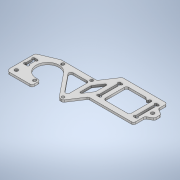
# Autodesk Inventor part: Ankle_side_frame
Saved by Autodesk Inventor 2020.4 (Build 244396000, 396)
## iProperties
Part Number: Ankle_side_frame
Material: アルミニウム 2014-T4
Document SubType Name: Modeling
Designer: Masato Kubotera
Density: 2.8 g/cm^3
Appearance: 滑らか - 淡い灰色
Description: A2017 T2
Mass: 9.74724 g
Surface Area: 49.2982 cm^2
Volume: 3.48116 cm^3
Author: Masato Kubotera
Autodesk Inventor part; units mm, degrees
ref_plane "YZ Plane" through (0, 0, 0) normal (1, 0, 0) x (0, 1, 0)
ref_plane "XZ Plane" through (0, 0, 0) normal (0, 1, 0) x (-1, 0, 0)
ref_plane "XY Plane" through (0, 0, 0) normal (0, 0, 1) x (1, 0, 0)
sketch "スケッチ1" plane through (0, 0, 0) normal (0, 0, 1) x (1, 0, 0)
  line L0 (28, 13.5) -> (1, 13.5) construction
  line L1 (1, 13.5) -> (1, -13.5) construction
  line L2 (1, -13.5) -> (28, -13.5) construction
  line L3 (28, -13.5) -> (28, 13.5) construction
  line L4 (28, 13.5) -> (1, -13.5) construction
  line L5 (1, 13.5) -> (28, -13.5) construction
  circle A0 centre (0, 0) radius 10.5 construction
  arc A1 (0, 16) -> (-12, 10.583) centre (0, 0) ccw construction
  line L6 (1, 0) -> (28, 0) construction
  line L7 (14.5, 13.5) -> (14.5, -13.5) construction
  circle A2 centre (28, 13.5) radius 1.35
  arc A3 (-0.35, 13) -> (2.35, 13) centre (1, 13) ccw
  line L8 (2.35, 13.5) -> (2.35, 13)
  line L9 (-0.35, 13.5) -> (-0.35, 13)
  arc A4 (2.35, 13.5) -> (-0.35, 13.5) centre (1, 13.5) ccw
  line L10 (-12, 10.583) -> (-12, -10.583) construction
  arc A5 (-12, -10.583) -> (0, -16) centre (0, 0) ccw construction
  circle A6 centre (28, -13.5) radius 1.35
  line L11 (-17.5, 5) -> (-14.5, 5) construction
  line L12 (-14.5, 5) -> (-14.5, -5) construction
  line L13 (-14.5, -5) -> (-17.5, -5) construction
  line L14 (-17.5, -5) -> (-17.5, 5) construction
  line L15 (-17.5, 5) -> (-14.5, -5) construction
  line L16 (-14.5, 5) -> (-17.5, -5) construction
  line L17 (-17.525, 5.025) -> (-14.475, 5.025)
  line L18 (-14.475, 5.025) -> (-14.475, 2.925) construction
  line L19 (-14.475, -5.025) -> (-17.525, -5.025)
  line L20 (-17.525, -5.025) -> (-17.525, -2.925) construction
  line L21 (-17.525, 5.025) -> (-14.475, -5.025) construction
  line L22 (-14.475, 5.025) -> (-17.525, -5.025) construction
  arc A7 (-17.525, 5.025) -> (-17.525, 2.925) centre (-17.525, 3.975) ccw
  line L23 (-17.5, 0) -> (-14.5, 0) construction
  line L24 (-16, 5) -> (-16, -5) construction
  arc A8 (-14.475, 2.925) -> (-14.475, 5.025) centre (-14.475, 3.975) ccw
  arc A9 (-17.525, -2.925) -> (-17.525, -5.025) centre (-17.525, -3.975) ccw
  arc A10 (-14.475, -5.025) -> (-14.475, -2.925) centre (-14.475, -3.975) ccw
  line L25 (-17.525, 2.925) -> (-17.525, 5.025) construction
  line L26 (-17.525, -2.925) -> (-17.525, 2.925)
  line L27 (-14.475, -2.925) -> (-14.475, -5.025) construction
  line L28 (-14.475, 2.925) -> (-14.475, -2.925)
  line L29 (-20.5, 8.739) -> (-20.5, -15.7058)
  line L30 (-3.2261, 16) -> (30.4, 16)
  line L31 (12.8981, 11.1) -> (26, 11.1)
  circle A11 centre (28, 13.5) radius 2.4 construction
  circle A12 centre (28, -13.5) radius 2.4 construction
  circle A13 centre (83.5, 15.5) radius 1.6
  line L32 (83.5, 12.0359) -> (80.5, 13.7679) construction
  line L33 (80.5, 13.7679) -> (80.5, 17.2321) construction
  line L34 (80.5, 17.2321) -> (83.5, 18.9641) construction
  line L35 (83.5, 18.9641) -> (86.5, 17.2321) construction
  line L36 (86.5, 17.2321) -> (86.5, 13.7679) construction
  line L37 (86.5, 13.7679) -> (83.5, 12.0359) construction
  line L38 (40, 30.4) -> (82.5, 30.4)
  line L39 (82.5, 30.4) -> (82.5, 21.8509)
  line L40 (82.5, 21.8509) -> (88.5, 18.3868)
  line L41 (88.5, 18.3868) -> (88.5, 12.6132)
  line L42 (88.5, 12.6132) -> (82.5, 9.1491)
  line L43 (82.5, 9.1491) -> (82.5, -1.4)
  line L44 (82.5, -1.4) -> (40, -1.4)
  line L45 (30.4, -16) -> (40, -1.4)
  line L46 (40, 30.4) -> (40, -1.4) construction
  line L47 (32, 8.9311) -> (32, -1.125)
  line L48 (33.8356, -1.6744) -> (38.8356, 5.9298)
  line L49 (39, 6.4792) -> (39, 16.4316)
  line L50 (37.1679, 16.9863) -> (32.1679, 9.4858)
  line L51 (-17.5, 10) -> (-14.5, 10) construction
  line L52 (-14.5, -10) -> (-17.5, -10) construction
  line L53 (-17.5, 10) -> (-14.5, -10) construction
  line L54 (-14.5, 10) -> (-17.5, -10) construction
  line L55 (40, 30.4) -> (30.4, 16)
  line L56 (30.4, 16) -> (30.4, -16) construction
  line L57 (43, 25.4) -> (45, 25.4) construction
  line L58 (45, 25.4) -> (45, 3.6) construction
  line L59 (45, 3.6) -> (43, 3.6) construction
  line L60 (43, 3.6) -> (43, 25.4) construction
  line L61 (43, 25.4) -> (45, 3.6) construction
  line L62 (45, 25.4) -> (43, 3.6) construction
  line L63 (42.975, 25.425) -> (45.025, 25.425)
  line L64 (45.025, 25.425) -> (45.025, 23.325) construction
  line L65 (45.025, 3.575) -> (42.975, 3.575)
  line L66 (42.975, 3.575) -> (42.975, 5.675) construction
  line L67 (42.975, 25.425) -> (45.025, 3.575) construction
  line L68 (45.025, 25.425) -> (42.975, 3.575) construction
  line L69 (44, 25.4) -> (44, 3.6) construction
  line L70 (43, 14.5) -> (45, 14.5) construction
  arc A14 (42.975, 25.425) -> (42.975, 23.325) centre (42.975, 24.375) ccw
  arc A15 (45.025, 23.325) -> (45.025, 25.425) centre (45.025, 24.375) ccw
  arc A16 (42.975, 5.675) -> (42.975, 3.575) centre (42.975, 4.625) ccw
  arc A17 (45.025, 3.575) -> (45.025, 5.675) centre (45.025, 4.625) ccw
  line L71 (45.025, 23.325) -> (45.025, 5.675)
  line L72 (42.975, 5.675) -> (42.975, 23.325)
  line L73 (45.025, 5.675) -> (45.025, 3.575) construction
  line L74 (28, 9.1) -> (28, -7.0627)
  arc A18 (8.3509, 6.7694) -> (-10.75, 0) centre (0, 0) ccw
  line L75 (8.3509, 6.7694) -> (26.0579, -15.0743)
  arc A19 (26.0579, -15.0743) -> (28, -16) centre (28, -13.5) ccw
  line L76 (11.3445, 7.8406) -> (24.4463, -8.3221)
  line L77 (-20.5, 8.739) -> (-3.2261, 16)
  line L78 (-20.5, -15.7058) -> (-18.8868, -18.5)
  line L79 (-14.2679, -16.5) -> (-17.7321, -16.5) construction
  line L80 (-17.7321, -16.5) -> (-19.4641, -13.5) construction
  line L81 (-19.4641, -13.5) -> (-17.7321, -10.5) construction
  line L82 (-17.7321, -10.5) -> (-14.2679, -10.5)
  line L83 (-14.2679, -10.5) -> (-12.5359, -13.5) construction
  line L84 (-12.5359, -13.5) -> (-14.2679, -16.5) construction
  line L85 (3.75, -18.5) -> (-18.8868, -18.5)
  circle A20 centre (-16, -13.5) radius 1.6
  line L86 (28, -16) -> (30.4, -16)
  line L87 (0, -16) -> (30.4, -16) construction
  arc A21 (24.4463, -8.3221) -> (28, -7.0627) centre (26, -7.0627) ccw
  arc A22 (2.35, -13) -> (-0.35, -13) centre (1, -13) ccw
  line L88 (-0.35, -13.5) -> (-0.35, -13)
  arc A23 (-0.35, -13.5) -> (2.35, -13.5) centre (1, -13.5) ccw
  line L89 (2.35, -13.5) -> (2.35, -13)
  arc A24 (-10.75, 0) -> (0, -10.75) centre (0, 0) ccw
  line L90 (0, -10.75) -> (3.75, -10.75)
  line L91 (3.75, -10.75) -> (3.75, -18.5)
  circle A25 centre (1, -13.5) radius 2.75 construction
  line L92 (73.5, 24.4) -> (73.5, 5.6)
  line L93 (71.5, 3.6) -> (51, 3.6)
  line L94 (49, 5.6) -> (49, 23.4)
  arc A26 (51, 25.4) -> (49, 23.4) centre (51, 23.4) ccw
  arc A27 (49, 5.6) -> (51, 3.6) centre (51, 5.6) ccw
  arc A28 (71.5, 3.6) -> (73.5, 5.6) centre (71.5, 5.6) ccw
  line L95 (42.975, 23.325) -> (42.975, 25.425) construction
  line L96 (77.5, 25.4) -> (79.5, 25.4) construction
  line L97 (79.5, 25.4) -> (79.5, 3.6) construction
  line L98 (77.475, 5.675) -> (77.475, 23.325)
  line L99 (78.5, 25.4) -> (78.5, 3.6) construction
  line L100 (79.5, 25.4) -> (77.5, 3.6) construction
  line L101 (77.5, 3.6) -> (77.5, 25.4) construction
  line L102 (77.5, 25.4) -> (79.5, 3.6) construction
  line L103 (79.525, 25.425) -> (77.475, 3.575) construction
  line L104 (77.475, 25.425) -> (79.525, 3.575) construction
  line L105 (79.5, 3.6) -> (77.5, 3.6) construction
  line L106 (79.525, 3.575) -> (77.475, 3.575)
  line L107 (77.475, 3.575) -> (77.475, 5.675) construction
  line L108 (79.525, 23.325) -> (79.525, 5.675)
  line L109 (79.525, 25.425) -> (79.525, 23.325) construction
  line L110 (77.475, 25.425) -> (79.525, 25.425)
  arc A29 (79.525, 3.575) -> (79.525, 5.675) centre (79.525, 4.625) ccw
  line L111 (79.525, 5.675) -> (79.525, 3.575) construction
  arc A30 (77.475, 5.675) -> (77.475, 3.575) centre (77.475, 4.625) ccw
  arc A31 (79.525, 23.325) -> (79.525, 25.425) centre (79.525, 24.375) ccw
  line L112 (77.5, 14.5) -> (79.5, 14.5) construction
  line L113 (77.475, 23.325) -> (77.475, 25.425) construction
  arc A32 (77.475, 25.425) -> (77.475, 23.325) centre (77.475, 24.375) ccw
  arc A33 (38.8356, 5.9298) -> (39, 6.4792) centre (38, 6.4792) ccw
  arc A34 (39, 16.4316) -> (37.1679, 16.9863) centre (38, 16.4316) ccw
  arc A35 (32.1679, 9.4858) -> (32, 8.9311) centre (33, 8.9311) ccw
  arc A36 (32, -1.125) -> (33.8356, -1.6744) centre (33, -1.125) ccw
  line L114 (30.4, 0) -> (40, 14.5) construction
  arc A37 (12.8981, 11.1) -> (11.3445, 7.8406) centre (12.8981, 9.1) ccw
  arc A38 (28, 9.1) -> (26, 11.1) centre (26, 9.1) ccw
  line L115 (71, 24.4) -> (71, 24.4)
  line L116 (69.2929, 23.6929) -> (68.1716, 24.8142)
  line L117 (51, 25.4) -> (66.7574, 25.4)
  line L118 (72, 25.4) -> (72.5, 25.4)
  arc A39 (72, 25.4) -> (71, 24.4) centre (72, 24.4) ccw
  arc A40 (73.5, 24.4) -> (72.5, 25.4) centre (72.5, 24.4) ccw
  arc A41 (69.2929, 23.6929) -> (71, 24.4) centre (70, 24.4) ccw
  arc A42 (68.1716, 24.8142) -> (66.7574, 25.4) centre (66.7574, 23.4) ccw
  point P0 (14.5, 0)
  point P1 (-16, 0)
  point P2 (-16, 0)
  point P3 (8.7023, 11.1)
  point P4 (28, 11.1)
  point P5 (32, 9.2339)
  point P6 (32, -4.4659)
  point P7 (39, 6.1799)
  point P8 (39, 19.7346)
  point P9 (44, 14.5)
  point P10 (-16, 0)
  point P11 (73.5, 25.4)
  point P12 (78.5, 14.5)
  point P13 (67.5858, 25.4)
  point P14 (71, 23.4)
  point P15 (71, 24.4)
  dimension "d0" = 27
  dimension "d1" = 27
  dimension "d2" = 21
  dimension "d6" = 2.7
  dimension "d9" = 0.5
  dimension "d10" = 1.35
  dimension "d11" = 1
  dimension "d12" = 16
  dimension "d13" = 12
  dimension "d14" = 3
  dimension "d16" = 2.5
  dimension "d18" = 0.025
  dimension "d28" = 3
  dimension "d29" = 4.8
  dimension "d53" = 4.8
  dimension "d54" = 10
  dimension "d55" = 0.025
  dimension "d56" = 1.05
  dimension "d80" = 3.2
  dimension "d87" = 2
  dimension "d88" = 2
  dimension "d90" = 2
  dimension "d91" = 6
  dimension "d109" = 5
  dimension "d113" = 1.05
  dimension "d118" = 45
  dimension "d120" = 4
  dimension "d121" = 4
  dimension "d122" = 3
  dimension "d124" = 14.5
  dimension "d135" = 17
  dimension "d136" = 20
  dimension "d141" = 0.25
  dimension "d143" = 3
  dimension "d144" = 6
  dimension "d145" = 2
  dimension "d146" = 2
  dimension "d148" = 0.5
  dimension "d149" = 3.2
  dimension "d151" = 2
  dimension "d153" = 5.5
  dimension "d154" = 2
  dimension "d158" = 21.8
  dimension "d159" = 0.025
  dimension "d160" = 5
  dimension "d171" = 2
  dimension "d173" = 4
  dimension "d175" = 0.025
  dimension "d178" = 34.5
  dimension "d183" = 4
  dimension "d184" = 1
  dimension "d185" = 3
  dimension "d186" = 1
  dimension "d187" = 1
  dimension "d188" = 5
  dimension "d189" = 2
  dimension "d191" = 1
  dimension "d192" = 45
  dimension "d194" = 2.5
  dimension "d197" = 1
  dimension "d198" = 2
  dimension "d199" = 2
  constraints: 240 end point, 70 point on circle, 43 centre point, 42 tangent, 37 parallel, 36 midpoint, 33 point on line, 20 symmetric about line, 17 perpendicular, 14 horizontal, 11 coincident, 7 equal radius, 6 vertical, 4 collinear, 1 concentric, 81 other
  measures "d0" distance of L2.end L1.end
  measures "d1" distance of L1.end L0.end
  measures "d2" diameter of A0
  measures "d6" diameter of A2
  measures "d9" distance of A3.centre L0.end
  measures "d10" radius of A4
  measures "d11" distance of point (0, 0) L6.start
  measures "d12" radius of A1
  measures "d13" distance from line of L10 A0.centre
  measures "d14" distance of L12.end L13.end
  measures "d16" distance between parallel lines of L10 L12
  measures "d18" distance between parallel lines of L17 L11
  measures "d28" distance between parallel lines of L29 L14
  measures "d29" diameter of A11
  measures "d53" diameter of A12
  measures "d54" distance between parallel lines of L13 L11
  measures "d55" distance between parallel lines of L14 L25
  measures "d56" radius of A7
  measures "d80" diameter of A13
  measures "d87" distance between parallel lines of L41 L36
  measures "d88" distance between parallel lines of L40 L35
  measures "d90" distance between parallel lines of L42 L37
  measures "d91" distance between parallel lines of L37 L34
  measures "d109" distance between parallel lines of L11 L51
  measures "d113" radius of A14
  measures "d118" distance from line of L58 point (0, 0)
  measures "d120" distance between parallel lines of L74 L47
  measures "d121" distance between parallel lines of L60 L49
  measures "d122" distance between parallel lines of L46 L60
  measures "d124" distance between parallel lines of L6 L70
  measures "d135" distance from line of point (-16, 0) L1
  measures "d136" distance between parallel lines of L52 L51
  measures "d141" radial gap between concentric circles of A18 A0
  measures "d143" distance between parallel lines of L75 L76
  measures "d144" distance between parallel lines of L79 L82
  measures "d145" distance between parallel lines of L78 L80
  measures "d146" distance between parallel lines of L85 L79
  measures "d148" distance between parallel lines of L82 L52
  measures "d149" diameter of A20
  measures "d151" radius of A21
  measures "d153" diameter of A25
  measures "d154" distance of L58.end L59.end
  measures "d158" distance between parallel lines of L59 L57
  measures "d159" distance between parallel lines of L57 L63
  measures "d160" distance between parallel lines of L44 L59
  measures "d171" radius of A26
  measures "d173" distance between parallel lines of L58 L94
  measures "d175" distance between parallel lines of L60 L95
  measures "d178" distance of L57.start L96.start
  measures "d183" distance between parallel lines of L92 L101
  measures "d184" distance from line of A13.centre L112
  measures "d185" distance between parallel lines of L39 L97
  measures "d186" distance between parallel lines of L97 L33
  measures "d187" radius of A33
  measures "d188" distance between parallel lines of L45 L48
  measures "d189" radius of A37
  measures "d191" radius of A39
  measures "d192" angle of L117 L116
  measures "d194" distance of L92.start L115.start
  measures "d197" radius of A41
  measures "d199" radius of A42
extrude "押し出し1" add sketch "スケッチ1" along normal blind 2
fillet "フィレット1" radius 2 16 edges at (-20.5, 8.739, 1) (-20.5, -15.7058, 1) (-18.8868, -18.5, 1) (30.4, 16, 1) (40, 30.4, 1) (82.5, 30.4, 1) (82.5, 21.8509, 1) (88.5, 18.3868, 1) (88.5, 12.6132, 1) (82.5, 9.1491, 1) (82.5, -1.4, 1) (40, -1.4, 1) (30.4, -16, 1) (-3.2261, 16, 1) (3.75, -18.5, 1) (3.75, -10.75, 1)
equation "\"d10\" = 0.5 * d6"
